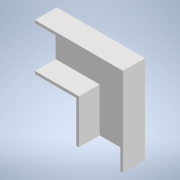
# Autodesk Inventor part: labik
Saved by Autodesk Inventor 2022 (Build 260153000, 153)
## iProperties
Created: 2024-07-28
Part Number: labik
Material: Типовые
Document SubType Name: Modeling
Designer: Капустяник Андрей
Density: 1 g/cm^3
Appearance: По умолчанию
Author: Капустяник Андрей
Autodesk Inventor part; units mm, degrees
ref_plane "YZ Plane" through (0, 0, 0) normal (1, 0, 0) x (0, 1, 0)
ref_plane "XZ Plane" through (0, 0, 0) normal (0, 1, 0) x (-1, 0, 0)
ref_plane "XY Plane" through (0, 0, 0) normal (0, 0, 1) x (1, 0, 0)
sketch "Эскиз1" plane through (0, 0, 0) normal (0, 0, 1) x (1, 0, 0)
  line L0 (150, 150) -> (-150, 150)
  line L1 (-150, 150) -> (-150, -150)
  line L2 (-150, -150) -> (150, -150)
  line L3 (150, -150) -> (150, 150)
  line L4 (150, 150) -> (-150, -150) construction
  line L5 (-150, 150) -> (150, -150) construction
  line L6 (-450, 150) -> (-150, 150)
  line L7 (-150, 150) -> (-150, -150)
  line L8 (-150, -150) -> (-450, -150)
  line L9 (-450, -150) -> (-450, 150)
  line L10 (-450, 150) -> (-150, -150) construction
  line L11 (-150, 150) -> (-450, -150) construction
  line L12 (150, -150) -> (-150, -150)
  line L13 (-150, -150) -> (-150, -450)
  line L14 (-150, -450) -> (150, -450)
  line L15 (150, -450) -> (150, -150)
  line L16 (150, -150) -> (-150, -450) construction
  line L17 (-150, -150) -> (150, -450) construction
  line L18 (170, 170) -> (-170, 170)
  line L19 (-170, 170) -> (-170, -170)
  line L20 (-170, -170) -> (170, -170)
  line L21 (170, -170) -> (170, 170)
  line L22 (170, -130) -> (-170, -130)
  line L23 (-170, -130) -> (-170, -470)
  line L24 (-170, -470) -> (170, -470)
  line L25 (170, -470) -> (170, -130)
  line L26 (-470, -170) -> (-130, -170)
  line L27 (-130, -170) -> (-130, 170)
  line L28 (-130, 170) -> (-470, 170)
  line L29 (-470, 170) -> (-470, -170)
  point P0 (0, 0)
  point P1 (-300, 0)
  point P2 (0, -300)
  point P3 (-170, 170)
  point P4 (170, -170)
  dimension "d0" = 300
  dimension "d1" = 300
  dimension "d2" = 300
  dimension "d3" = 300
  dimension "d4" = 300
  dimension "d5" = 300
  dimension "d6" = 20
  dimension "d7" = 20
  dimension "d8" = 20
  constraints: 60 end point, 12 parallel, 6 midpoint, 6 perpendicular, 4 collinear, 3 horizontal, 9 other
  measures "d0" distance of L2.end L1.end
  measures "d1" distance of L1.end L0.end
  measures "d2" distance of L7.end L8.end
  measures "d3" distance of L6.end L7.end
  measures "d4" distance of L14.end L13.end
  measures "d5" distance of L13.end L12.end
  measures "d6" distance between parallel lines of L3 L21
  measures "d7" distance between parallel lines of L15 L25
  measures "d8" distance between parallel lines of L8 L26
extrude "Выдавливание1" add sketch "Эскиз1" along normal blind 10
sketch "Эскиз2" plane through (0, 0, 10) normal (0, 0, 1) x (1, 0, 0)
  line L0 (170, 170) -> (-470, 170) projected
  line L1 (-470, 170) -> (-470, -170) projected
  line L2 (-470, -170) -> (-170, -170) projected
  line L3 (-170, -170) -> (-170, -470) projected
  line L4 (-170, -470) -> (170, -470) projected
  line L5 (170, -470) -> (170, 170) projected
  line L6 (150, 150) -> (-450, 150)
  line L7 (-450, 150) -> (-450, -150)
  line L8 (-450, -150) -> (-150, -150)
  line L9 (-150, -150) -> (-150, -450)
  line L10 (-150, -450) -> (150, -450)
  line L11 (150, -450) -> (150, 150)
  line L12 (-170, -470) -> (170, -470) projected
  line L13 (150, -450) -> (-150, -450)
  line L14 (-150, -450) -> (-150, -470)
  line L15 (-150, -470) -> (150, -470)
  line L16 (150, -470) -> (150, -450)
  line L17 (-470, 170) -> (-470, -170) projected
  line L18 (-450, 150) -> (-470, 150)
  line L19 (-470, 150) -> (-470, -150)
  line L20 (-470, -150) -> (-450, -150)
  line L21 (-450, -150) -> (-450, 150)
  point P0 (0, 0)
  dimension "d11" = 20
  constraints: 28 end point, 4 parallel, 2 horizontal, 2 perpendicular, 2 point on line, 5 other
  measures "d11" distance between parallel lines of L5 L11
extrude "Выдавливание2" add sketch "Эскиз2" along normal blind 150 contours L5 L4 L16 L11 L6 L18 L1 L0 | L20 L8 L9 L14 L4 L3 L2 L1
